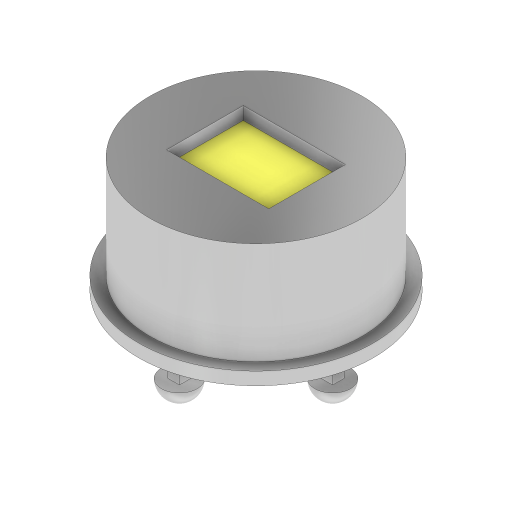
# Autodesk Inventor part: PIR sensor RE200B
Saved by Autodesk Inventor 2024 (Build 280153000, 153)
## iProperties
Created: 2024-09-23
Part Number: PIR sensor RE200B
Material: Generic
Document SubType Name: Modeling
Designer: Laith Al-Sadi
Density: 1 g/cm^3
Appearance: Chrome - Polished
Author: Laith Al-Sadi
Autodesk Inventor part; units mm, degrees
ref_plane "YZ Plane" through (0, 0, 0) normal (1, 0, 0) x (0, 1, 0)
ref_plane "XZ Plane" through (0, 0, 0) normal (0, 1, 0) x (-1, 0, 0)
sketch "Sketch1" plane through (0, 0, 0) normal (0, 0, 1) x (1, 0, 0)
  line L0 (0, 4.5) -> (4.15, 4.5)
  line L1 (4.15, 4.5) -> (4.15, 0.5)
  line L2 (4.6, 0) -> (0, 0)
  line L3 (0, 0) -> (0, 4.5)
  line L4 (4.6, 0) -> (4.6, 0.5)
  line L5 (4.6, 0.5) -> (4.15, 0.5)
  dimension "d0" = 4.15
  dimension "d2" = 0.5
  dimension "d3" = 4.6
  dimension "d5" = 4.5
  constraints: 12 end point, 4 perpendicular, 1 horizontal, 1 vertical
  measures "d0" distance of L0.start L0.end
  measures "d2" distance of L2.start L4.end
  measures "d3" distance between parallel lines of L3 L4
  measures "d5" distance between parallel lines of L0 L2
revolve "Revolution1" add sketch "Sketch1" angle 360 about axis through (0, 0, 0) along (0, 1, 0)
sketch "Sketch2" plane through (0, 4.5, 0) normal (0, 1, 0) x (1, 0, 0)
  line L0 (-2, 1.5) -> (2, 1.5)
  line L1 (2, 1.5) -> (2, -1.5)
  line L2 (2, -1.5) -> (-2, -1.5)
  line L3 (-2, -1.5) -> (-2, 1.5)
  line L4 (-2, 1.5) -> (2, -1.5) construction
  line L5 (2, 1.5) -> (-2, -1.5) construction
  point P0 (0, 0)
  dimension "d7" = 4
  dimension "d8" = 3
  constraints: 12 end point, 2 midpoint, 2 parallel, 1 horizontal, 1 perpendicular
  measures "d7" distance of L0.start L0.end
  measures "d8" distance of L0.end L1.end
extrude "Extrusion1" cut sketch "Sketch2" against normal blind 0.5
sketch "Sketch3" plane through (0, 0, 0) normal (0, -1, 0) x (1, 0, 0)
  line L0 (-0.225, 0.225) -> (0.225, 0.225)
  line L1 (0.225, 0.225) -> (0.225, -0.225)
  line L2 (0.225, -0.225) -> (-0.225, -0.225)
  line L3 (-0.225, -0.225) -> (-0.225, 0.225)
  line L4 (-0.225, 0.225) -> (0.225, -0.225) construction
  line L5 (0.225, 0.225) -> (-0.225, -0.225) construction
  line L6 (2.775, 0.225) -> (3.225, 0.225)
  line L7 (3.225, 0.225) -> (3.225, -0.225)
  line L8 (3.225, -0.225) -> (2.775, -0.225)
  line L9 (2.775, -0.225) -> (2.775, 0.225)
  line L10 (2.775, 0.225) -> (3.225, -0.225) construction
  line L11 (3.225, 0.225) -> (2.775, -0.225) construction
  line L12 (-3.225, 0.225) -> (-2.775, 0.225)
  line L13 (-2.775, 0.225) -> (-2.775, -0.225)
  line L14 (-2.775, -0.225) -> (-3.225, -0.225)
  line L15 (-3.225, -0.225) -> (-3.225, 0.225)
  line L16 (-3.225, 0.225) -> (-2.775, -0.225) construction
  line L17 (-2.775, 0.225) -> (-3.225, -0.225) construction
  line L18 (-0.225, 0.225) -> (0.225, 0.225)
  line L19 (0.225, 0.225) -> (0.225, -0.225)
  line L20 (0.225, -0.225) -> (-0.225, -0.225)
  line L21 (-0.225, -0.225) -> (-0.225, 0.225)
  line L22 (-0.225, 0.225) -> (0.225, -0.225) construction
  line L23 (0.225, 0.225) -> (-0.225, -0.225) construction
  line L24 (-0.225, 3.225) -> (0.225, 3.225)
  line L25 (0.225, 3.225) -> (0.225, 2.775)
  line L26 (0.225, 2.775) -> (-0.225, 2.775)
  line L27 (-0.225, 2.775) -> (-0.225, 3.225)
  line L28 (-0.225, 3.225) -> (0.225, 2.775) construction
  line L29 (0.225, 3.225) -> (-0.225, 2.775) construction
  point P0 (0, 0)
  point P1 (3, 0)
  point P2 (-3, 0)
  point P3 (0, 0)
  point P4 (0, 3)
  point P5 (0, 0)
  point P6 (0, 0)
  dimension "d11" = 0.45
  dimension "d12" = 0.45
  dimension "d15" = 3
  dimension "d18" = 3
  dimension "d26" = 0.45
  dimension "d27" = 0.45
  dimension "d28" = 3
  constraints: 60 end point, 6 midpoint, 4 horizontal, 4 parallel, 2 collinear, 2 perpendicular, 1 vertical alignment, 31 other
  measures "d11" distance of L0.start L0.end
  measures "d12" distance of L0.end L1.end
  measures "d15" distance of point (0, 0) point (3, 0)
  measures "d18" distance of point (0, 0) point (-3, 0)
  measures "d26" distance of L25.end L26.end
  measures "d27" distance of L24.end L25.end
  measures "d28" distance of point (0, 0) point (0, 3)
extrude "Extrusion2" add sketch "Sketch3" along normal blind 2 contours L6 L7 L8 L9 | L12 L13 L14 L15 | L24 L25 L26 L27
sketch "Sketch4" plane through (0, 0, 0) normal (0, -1, 0) x (1, 0, 0)
  line L0 (0, 0) -> (-4.5837, -4.5837)
  line L1 (0, 0) -> (-2.6627, 0)
  circle A0 centre (0, 0) radius 4.6 projected
  line L2 (-3.0336, -3.4579) -> (-3.4579, -3.8822)
  line L3 (-3.4579, -3.8822) -> (-3.8822, -3.4579)
  line L4 (-3.8822, -3.4579) -> (-3.4579, -3.0336)
  point P0 (-3.67, -3.67)
  dimension "d29" = 45
  dimension "d30" = 0.6
  dimension "d31" = 0.6
  constraints: 10 end point, 2 perpendicular, 2 point on circle, 1 horizontal, 1 midpoint, 1 parallel, 1 point on line
  measures "d29" angle of L1 L0
  measures "d30" distance of L2.end L3.end
  measures "d31" distance of L3.end L4.end
extrude "Extrusion3" add sketch "Sketch4" against normal up to surface (0.5 mm away) contours A0 L2 L3 L0 | L0 L3 L4 A0
ref_plane "Work Plane1" through (-3, 0, -0.225) normal (-1, 0, 0) x (0, 0, 1)
sketch "Sketch6" plane through (-3, 0, -0.225) normal (-1, 0, 0) x (0, 0, 1)
  arc A0 (-0.475, -1.5) -> (0.225, -2.2) centre (0.225, -1.5) ccw
  line L0 (0, -2) -> (0.45, -2) projected
  line L1 (-0.475, -1.5) -> (0.225, -1.5)
  line L2 (0.225, -1.5) -> (0.225, -2.2)
  point P0 (0.225, 0)
  point P1 (0.225, -2)
  dimension "d36" = 0.5
  dimension "d37" = 0.7
  constraints: 4 end point, 2 point on circle, 2 vertical alignment, 1 centre point, 1 horizontal, 1 horizontal alignment, 1 midpoint, 1 perpendicular
  measures "d36" distance from line of L0 L1.end
  measures "d37" radius of A0
revolve "Revolution2" add sketch "Sketch6" angle 360 about axis through (-3, -1.5, 0) along (0, -1, 0)
pattern_circular "Circular Pattern1" count 3 over 180 about axis through (0, 2.5, 0) along (0, 1, 0) of "Revolution2"
body "Solid1"
